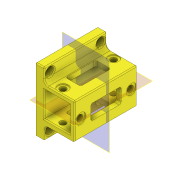
# Autodesk Inventor part: Part3
Saved by Autodesk Inventor 2021 (Build 250183000, 183)
## iProperties
Created: 2021-02-20
Part Number: Part3
Material: Generic
Document SubType Name: Modeling
Designer: dsdan
Density: 1 g/cm^3
Appearance: Default
Author: dsdan
Autodesk Inventor part; units mm, degrees
ref_plane "YZ Plane" through (0, 0, 0) normal (1, 0, 0) x (0, 1, 0)
ref_plane "XZ Plane" through (0, 0, 0) normal (0, 1, 0) x (-1, 0, 0)
ref_plane "XY Plane" through (0, 0, 0) normal (0, 0, 1) x (1, 0, 0)
sketch "Sketch1" plane through (0, 0, 0) normal (0, 0, 1) x (1, 0, 0)
  line L0 (-21.4968, -47.8892) -> (-21.4968, 25.0724)
  circle A0 centre (0, -16.4084) radius 3 construction
  arc A1 (-5.4102, -9.5755) -> (5.4102, -9.5755) centre (0, 0) ccw construction
  line L1 (-5.4102, -9.5755) -> (-5.4102, -5.6134) construction
  line L2 (-5.4102, -5.6134) -> (-3.7592, -5.6134) construction
  line L3 (-3.7592, -5.6134) -> (-3.2512, -5.1054) construction
  line L4 (-3.2512, -5.1054) -> (-3.2512, -3.9116) construction
  line L5 (-3.2512, -3.9116) -> (-11.4808, -3.9116) construction
  line L6 (-11.4808, -3.9116) -> (-12.4968, -4.9276) construction
  line L7 (-12.4968, -4.9276) -> (-12.4968, -13.1572) construction
  line L8 (-12.4968, -13.1572) -> (-11.303, -13.1572) construction
  line L9 (-11.303, -13.1572) -> (-10.795, -12.6492) construction
  line L10 (-10.795, -12.6492) -> (-10.795, -11.0109) construction
  line L11 (-10.795, -11.0109) -> (-6.8257, -11.0109) construction
  arc A2 (-6.8257, -21.8059) -> (-6.8257, -11.0109) centre (-16.4084, -16.4084) ccw construction
  line L12 (-6.8257, -21.8059) -> (-10.795, -21.8059) construction
  line L13 (-10.795, -21.8059) -> (-10.795, -20.1676) construction
  line L14 (-10.795, -20.1676) -> (-11.303, -19.6596) construction
  line L15 (-11.303, -19.6596) -> (-12.4968, -19.6596) construction
  line L16 (-12.4968, -19.6596) -> (-12.4968, -27.8892) construction
  line L17 (-12.4968, -27.8892) -> (-11.4808, -28.9052) construction
  line L18 (-11.4808, -28.9052) -> (-3.2512, -28.9052) construction
  line L19 (-3.2512, -28.9052) -> (-3.2512, -27.7114) construction
  line L20 (-3.2512, -27.7114) -> (-3.7592, -27.2034) construction
  line L21 (-3.7592, -27.2034) -> (-5.4102, -27.2034) construction
  line L22 (-5.4102, -27.2034) -> (-5.4102, -23.2413) construction
  arc A3 (5.4102, -23.2413) -> (-5.4102, -23.2413) centre (0, -32.8168) ccw construction
  line L23 (5.4102, -23.2413) -> (5.4102, -27.2034) construction
  line L24 (5.4102, -27.2034) -> (3.7592, -27.2034) construction
  line L25 (3.7592, -27.2034) -> (3.2512, -27.7114) construction
  line L26 (3.2512, -27.7114) -> (3.2512, -28.9052) construction
  line L27 (3.2512, -28.9052) -> (11.4808, -28.9052) construction
  line L28 (11.4808, -28.9052) -> (12.4968, -27.8892) construction
  line L29 (12.4968, -27.8892) -> (12.4968, -19.6596) construction
  line L30 (12.4968, -19.6596) -> (11.303, -19.6596) construction
  line L31 (11.303, -19.6596) -> (10.795, -20.1676) construction
  line L32 (10.795, -20.1676) -> (10.795, -21.8059) construction
  line L33 (10.795, -21.8059) -> (6.8257, -21.8059) construction
  arc A4 (6.8257, -11.0109) -> (6.8257, -21.8059) centre (16.4084, -16.4084) ccw construction
  line L34 (6.8257, -11.0109) -> (10.795, -11.0109) construction
  line L35 (10.795, -11.0109) -> (10.795, -12.6492) construction
  line L36 (10.795, -12.6492) -> (11.303, -13.1572) construction
  line L37 (11.303, -13.1572) -> (12.4968, -13.1572) construction
  line L38 (12.4968, -13.1572) -> (12.4968, -4.9276) construction
  line L39 (12.4968, -4.9276) -> (11.4808, -3.9116) construction
  line L40 (11.4808, -3.9116) -> (3.2512, -3.9116) construction
  line L41 (3.2512, -3.9116) -> (3.2512, -5.1054) construction
  line L42 (3.2512, -5.1054) -> (3.7592, -5.6134) construction
  line L43 (3.7592, -5.6134) -> (5.4102, -5.6134) construction
  line L44 (5.4102, -5.6134) -> (5.4102, -9.5755) construction
  circle A5 centre (-8.4963, -7.9121) radius 2.0193 construction
  circle A6 centre (8.4963, -24.9047) radius 2.0193 construction
  circle A7 centre (0, -16.4084) radius 3 construction
  circle A8 centre (-8.4963, -24.9047) radius 2.0193 construction
  circle A9 centre (8.4963, -7.9121) radius 2.0193 construction
  line L45 (-21.4968, -47.8892) -> (-12.4968, -47.8892)
  line L46 (-12.4968, -47.8892) -> (-12.4968, -37.9052)
  line L47 (-12.4968, 5.0884) -> (-12.4968, 15.0724)
  line L48 (-12.4968, 15.0724) -> (-21.4968, 15.0724)
  line L49 (-12.4968, -19.6596) -> (-12.4968, -13.1572) construction
  line L50 (-8.4968, -33.9052) -> (17.4968, -33.9052)
  line L51 (17.4968, 1.0884) -> (-8.4968, 1.0884)
  line L52 (3.2512, -28.9052) -> (-3.2512, -28.9052) construction
  line L53 (3.2512, -3.9116) -> (-3.2512, -3.9116) construction
  arc A10 (-8.4968, -33.9052) -> (-12.4968, -37.9052) centre (-8.4968, -37.9052) ccw
  arc A11 (-12.4968, 5.0884) -> (-8.4968, 1.0884) centre (-8.4968, 5.0884) ccw
  line L54 (17.4968, -33.9052) -> (17.4968, 1.0884)
  line L55 (11.4808, -28.9052) -> (12.4968, -28.9052) construction
  line L56 (12.4968, -28.9052) -> (12.4968, -3.9116) construction
  line L57 (12.4968, -3.9116) -> (11.4808, -3.9116) construction
  line L58 (-12.5218, -3.8866) -> (-12.5218, -28.9302)
  line L59 (-12.5218, -28.9302) -> (12.5218, -28.9302)
  line L60 (12.5218, -28.9302) -> (12.5218, -3.8866)
  line L61 (12.5218, -3.8866) -> (-12.5218, -3.8866)
  line L62 (-12.5218, -3.8866) -> (12.5218, -28.9302) construction
  line L63 (-12.5218, -28.9302) -> (12.5218, -3.8866) construction
  dimension "d0" = 20
  dimension "d1" = 20
  dimension "d3" = 5
  dimension "d4" = 5
  dimension "d6" = 4
  dimension "d30" = 5
  dimension "d45" = 9
  dimension "d61" = 0.025
  dimension "d62" = 0.025
  constraints: 41 end point, 6 perpendicular, 5 point on line, 4 point on circle, 4 tangent, 3 collinear, 3 horizontal, 3 parallel, 2 centre point, 2 midpoint, 2 vertical, 1 equal radius
  measures "d0" distance of L6.end L47.end
  measures "d1" distance of L45.end L16.end
  measures "d3" distance between parallel lines of L27 L50
  measures "d4" vertical distance of L39.end L51.start
  measures "d6" radius of A10
  measures "d30" distance between parallel lines of L29 L54
  measures "d45" distance between parallel lines of L47 L0
  measures "d61" distance between parallel lines of L29 L60
  measures "d62" distance between parallel lines of L18 L59
extrude "Extrusion1" add sketch "Sketch1" against normal blind 62
sketch "Sketch2" plane through (17.4968, 4.0884, 0) normal (1, 0, 0) x (0, -1, 0)
  circle A0 centre (20.4968, 56) radius 5.1
  line L0 (37.9936, 0) -> (37.9936, 62) construction
  line L1 (3, 0) -> (37.9936, 62) construction
  line L2 (37.9936, 0) -> (3, 62) construction
  point P0 (3, 62)
  point P1 (20.4968, 31)
  point P2 (20.4968, 31)
  dimension "d9" = 10.2
  dimension "d54" = 25
  constraints: 4 end point, 2 midpoint, 1 centre point, 1 coincident, 1 vertical alignment
  measures "d9" diameter of A0
  measures "d54" distance of A0.centre point (20.497, 31)
extrude "Extrusion2" cut sketch "Sketch2" against normal blind 1 and the other way blind 1
sketch "Sketch3" plane through (16.4968, -16.4084, -56) normal (1, 0, 0) x (0, 0, -1)
  circle A0 centre (0, 0) radius 3.05
  circle A1 centre (0, 0) radius 5.1 projected
  point P0 (-56, 16.4084)
  point P1 (4.9808, -1.0962)
  dimension "d14" = 6.1
  constraints: 1 centre point, 2 other
  measures "d14" diameter of A0
extrude "Extrusion3" cut sketch "Sketch3" against normal blind 10 contours A0
sketch "Sketch4" plane through (-21.4968, -47.8892, 0) normal (-1, 0, 0) x (0, 0, 1)
  line L0 (0, 62.9616) -> (0, 0) projected
  line L1 (0, 0) -> (-62, 0) projected
  line L2 (-62, 0) -> (-62, 62.9616) projected
  circle A0 centre (-6, 6.4808) radius 3.05
  line L3 (0, 62.9616) -> (-62, 62.9616) projected
  line L4 (0, 0) -> (-62, 0) projected
  line L5 (-31, 0) -> (-31, 62.9616) construction
  line L6 (-62, 31.4808) -> (0, 31.4808) construction
  circle A1 centre (-56, 6.4808) radius 3.05
  circle A2 centre (-6, 56.4808) radius 3.05
  circle A3 centre (-56, 56.4808) radius 3.05
  point P0 (0, 47.8892)
  dimension "d21" = 6.1
  dimension "d35" = 25
  dimension "d36" = 25
  dimension "d39" = 50
  dimension "d42" = 50
  constraints: 4 centre point, 4 end point, 4 midpoint, 1 horizontal, 1 vertical, 6 other
  measures "d21" diameter of A0
  measures "d35" distance from line of L5 A0.centre
  measures "d36" distance from line of L6 A0.centre
  measures "d39" distance of A0.centre A1.centre
  measures "d42" distance of A0.centre A2.centre
extrude "Extrusion4" cut sketch "Sketch4" against normal through all contours A0 | A1 | A2 | A3
sketch "Sketch6" plane through (-12.4968, 6.5884, -8.2999) normal (1, 0, 0) x (0, 0, -1)
  circle A0 centre (47.7001, 2.0032) radius 3.05 projected
  circle A1 centre (47.7001, 2.0032) radius 4
  circle A2 centre (-2.2999, 2.0032) radius 3.05 projected
  circle A3 centre (-2.2999, 2.0032) radius 4
  circle A4 centre (-2.2999, -47.9968) radius 3.05 projected
  circle A5 centre (-2.2999, -47.9968) radius 4
  circle A6 centre (47.7001, -47.9968) radius 3.05 projected
  circle A7 centre (47.7001, -47.9968) radius 4
  point P0 (-8.2999, -6.5884)
  point P1 (50, -45.9936)
  dimension "d46" = 8
  dimension "d47" = 8
  dimension "d48" = 8
  dimension "d49" = 8
  constraints: 4 centre point, 4 coincident, 1 other
  measures "d46" diameter of A1
  measures "d47" diameter of A3
  measures "d48" diameter of A5
  measures "d49" diameter of A7
extrude "Extrusion6" cut sketch "Sketch6" along normal blind 5 and the other way blind 6 contours A0 | A1 | A2 | A3 | A4 | A5 | A6 | A7
ref_plane "Work Plane2" through (0, 0, -31) normal (0, 0, -1) x (-1, 0, 0)
mirror "Mirror2" about plane through (0, 0, -31) normal (0, 0, -1) of "Extrusion2", "Extrusion3"
sketch "Sketch9" plane through (17.4968, -33.9052, 0) normal (1, 0, 0) x (0, 0, -1)
  line L0 (18, 9.9968) -> (44, 9.9968)
  line L1 (46, 11.9968) -> (46, 22.9968)
  line L2 (44, 24.9968) -> (18, 24.9968)
  line L3 (16, 22.9968) -> (16, 11.9968)
  line L4 (16, 9.9968) -> (46, 24.9968) construction
  line L5 (46, 9.9968) -> (16, 24.9968) construction
  circle A0 centre (56, 17.4968) radius 3.05 projected
  circle A1 centre (6, 17.4968) radius 5.1 projected
  circle A2 centre (56, 17.4968) radius 5.1 projected
  line L6 (0, 0) -> (0, 34.9936) projected
  line L7 (0, 0) -> (62, 0) projected
  line L8 (62, 34.9936) -> (62, 0) projected
  line L9 (0, 34.9936) -> (62, 34.9936) projected
  arc A3 (46, 22.9968) -> (44, 24.9968) centre (44, 22.9968) ccw
  arc A4 (44, 9.9968) -> (46, 11.9968) centre (44, 11.9968) ccw
  arc A5 (16, 11.9968) -> (18, 9.9968) centre (18, 11.9968) ccw
  arc A6 (18, 24.9968) -> (16, 22.9968) centre (18, 22.9968) ccw
  point P0 (0, 33.9052)
  point P1 (31, 17.4968)
  point P2 (31, 17.4968)
  point P3 (31, 17.4968)
  point P4 (31, 34.9936)
  dimension "d55" = 15
  dimension "d56" = 30
  dimension "d57" = 2
  dimension "d58" = 2
  constraints: 12 end point, 8 point on circle, 8 point on line, 8 tangent, 5 midpoint, 4 centre point, 2 equal radius, 2 parallel, 1 horizontal, 1 horizontal alignment, 1 perpendicular, 1 vertical alignment
  measures "d55" distance between parallel lines of L2 L0
  measures "d56" distance of L4.start L5.start
  measures "d57" radius of A3
  measures "d58" radius of A6
extrude "Extrusion7" cut sketch "Sketch9" against normal up to surface (30.0186 mm away) contours A5 L3 A6 L2 A3 L1 A4 L0
chamfer "Chamfer1" distance 1 angle 45 23 edges at (-12.4968, 15.0724, -31) (-21.4968, 15.0724, -31) (-12.4968, -47.8892, -31) (-21.4968, -47.8892, -31) (-11.3252, 2.26, 0) (-12.4968, 10.0804, 0) (4.5, 1.0884, 0) (-16.9968, 15.0724, 0) (-16.9968, 15.0724, -62) (-21.4968, -16.4084, 0) (-21.4968, -16.4084, -62) (-12.4968, 10.0804, -62) (-11.3252, 2.26, -62) (4.5, 1.0884, -62) (4.5, -33.9052, -62) (-11.3252, -35.0768, -62) (-12.4968, -42.8972, -62) (-16.9968, -47.8892, -62) (-16.9968, -47.8892, 0) (17.4968, 1.0884, -31) (17.4968, -16.4084, -62) (17.4968, -33.9052, -31) (17.4968, -16.4084, 0)
chamfer "Chamfer2" distance 1 angle 45 12 edges at (-12.4658, 4.5916, -6) (-12.4968, 6.5572, -9.444) (-12.4968, 12.0356, -3.9656) (-12.4658, 4.5916, -56) (-12.4968, 6.5572, -59.444) (-12.4968, 12.0356, -53.9656) (-12.4968, -44.8524, -3.9656) (-12.4968, -39.374, -9.444) (-12.4658, -37.4084, -6) (-12.4968, -44.8524, -53.9656) (-12.4968, -39.374, -59.444) (-12.4658, -37.4084, -56)
sketch "Sketch10" plane through (-8.4968, 1.0884, -1) normal (0, 1, 0) x (1, 0, 0)
  circle A0 centre (8.4968, 5) radius 3.05
  circle A1 centre (8.4968, 55) radius 3.05
  line L0 (-4.025, -1) -> (21.0186, -1) projected
  line L1 (21.0186, 61) -> (-4.025, 61) projected
  line L2 (24.9936, 8.05) -> (24.9936, 1.95) projected
  line L3 (24.9936, 58.05) -> (24.9936, 51.95) projected
  point P0 (8.4968, -1)
  point P1 (8.4968, -1)
  point P2 (24.9936, 5)
  point P3 (24.9936, 55)
  dimension "d67" = 6.1
  constraints: 3 midpoint, 2 centre point, 2 horizontal alignment, 2 vertical alignment, 1 equal radius
  measures "d67" diameter of A1
extrude "Extrusion8" cut sketch "Sketch10" against normal through all
sketch "Sketch11" plane through (-8.4968, 1.0884, -1) normal (0, 1, 0) x (1, 0, 0)
  circle A0 centre (8.4968, 5) radius 3.05 projected
  circle A1 centre (8.4968, 5) radius 5.1
  circle A2 centre (8.4968, 55) radius 3.05 projected
  circle A3 centre (8.4968, 55) radius 5.1
  point P0 (8.4968, -1)
  dimension "d70" = 10.2
  dimension "d71" = 10.2
  constraints: 2 centre point, 2 coincident
  measures "d70" diameter of A1
  measures "d71" diameter of A3
extrude "Extrusion9" cut sketch "Sketch11" against normal blind 1
ref_plane "Work Plane3" through (-8.4968, -16.4084, -1) normal (0, 1, 0) x (1, 0, 0)
mirror "Mirror3" about plane through (-8.4968, -16.4084, -1) normal (0, 1, 0) of "Extrusion9"
chamfer "Chamfer3" distance 1 angle 45 8 edges at (0, -3.8866, 0) (12.5218, -16.4084, 0) (0, -28.9302, 0) (-12.5218, -16.4084, 0) (-12.5218, -16.4084, -62) (0, -28.9302, -62) (12.5218, -16.4084, -62) (0, -3.8866, -62)
sketch "Sketch12" plane through (-8.4968, 1.0884, -1) normal (0, 1, 0) x (1, 0, 0)
  line L0 (2.9968, 15) -> (13.9968, 15)
  line L1 (15.9968, 17) -> (15.9968, 43)
  line L2 (13.9968, 45) -> (2.9968, 45)
  line L3 (0.9968, 43) -> (0.9968, 17)
  line L4 (0.9968, 15) -> (15.9968, 45) construction
  line L5 (15.9968, 15) -> (0.9968, 45) construction
  arc A0 (15.9968, 43) -> (13.9968, 45) centre (13.9968, 43) ccw
  arc A1 (13.9968, 15) -> (15.9968, 17) centre (13.9968, 17) ccw
  arc A2 (0.9968, 17) -> (2.9968, 15) centre (2.9968, 17) ccw
  arc A3 (2.9968, 45) -> (0.9968, 43) centre (2.9968, 43) ccw
  circle A4 centre (8.4968, 5) radius 3.05 projected
  circle A5 centre (8.4968, 55) radius 3.05 projected
  point P0 (8.4968, -1)
  point P1 (8.4968, 30)
  point P2 (8.4968, 30)
  point P3 (8.4968, 30)
  dimension "d77" = 30
  dimension "d78" = 15
  dimension "d79" = 2
  dimension "d80" = 2
  dimension "d81" = 25
  dimension "d82" = 25
  constraints: 12 end point, 8 point on circle, 8 point on line, 8 tangent, 4 centre point, 4 midpoint, 2 equal radius, 2 parallel, 1 horizontal, 1 perpendicular, 1 vertical alignment
  measures "d77" distance between parallel lines of L2 L0
  measures "d78" distance of L4.start L5.start
  measures "d79" radius of A0
  measures "d80" radius of A3
  measures "d81" distance of point (8.497, 30) A4.centre
  measures "d82" distance of A5.centre point (8.497, 30)
extrude "Extrusion10" cut sketch "Sketch12" against normal through all contours A2 L3 A3 L2 A0 L1 A1 L0
equation "\"d1\" = d0"
equation "\"d3\" = d4"
equation "\"d30\" = d4"
equation "\"d81\" = d82"
body "Solid1"
